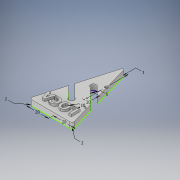
# Autodesk Inventor part: directional_arrow
Saved by Autodesk Inventor 2019 (Build 230136000, 136)
## iProperties
Created: 2019-04-03
Part Number: directional_arrow
Material: Generic
Document SubType Name: Modeling
Designer: jmc
Density: 1 g/cm^3
Appearance: Default
URL: https://www.amazon.es/MagiDeal-Marcador-Flecha-Triangular-Naufragios/dp/B07CHZN8H6
Author: jmc
Autodesk Inventor part; units mm, degrees
ref_plane "YZ Plane" through (0, 0, 0) normal (1, 0, 0) x (0, 1, 0)
ref_plane "XZ Plane" through (0, 0, 0) normal (0, 1, 0) x (-1, 0, 0)
ref_plane "XY Plane" through (0, 0, 0) normal (0, 0, 1) x (1, 0, 0)
sketch "Sketch1" plane through (0, 0, 0) normal (0, 1, 0) x (-1, 0, 0)
  line L0 (0, 0) -> (0, -40) construction
  line L1 (0, -40) -> (0, 29.0613) construction
  line L2 (0, 29.0613) -> (17.3386, 29.0613)
  line L3 (0, 29.0613) -> (-17.3386, 29.0613)
  arc A0 (19.2597, 26.505) -> (17.3386, 29.0613) centre (17.3386, 27.0613) ccw
  arc A1 (-17.3386, 29.0613) -> (-19.2597, 26.505) centre (-17.3386, 27.0613) ccw
  arc A2 (-0.9605, -36.6832) -> (0.9605, -36.6832) centre (0, -36.4051) ccw
  line L4 (0, 0) -> (0, 10) construction
  line L5 (0, 10) -> (0, -10) construction
  arc A3 (2.4749, 10.3536) -> (0, 7.5) centre (0, 10) ccw
  arc A4 (-1.7678, -11.7678) -> (0, -7.5) centre (0, -10) ccw
  line L6 (2.4749, 10.3536) -> (11.8634, 0.965)
  line L7 (-0.3536, 7.5251) -> (10.5931, -3.4215)
  line L8 (-1.7678, -11.7678) -> (-10.7883, -2.7472)
  line L9 (0.3536, -7.5251) -> (-13.3826, 6.211)
  line L10 (19.2597, 26.505) -> (11.8634, 0.965)
  line L11 (10.5931, -3.4215) -> (0.9605, -36.6832)
  line L12 (-19.2597, 26.505) -> (-13.3826, 6.211)
  line L13 (-10.7883, -2.7472) -> (-0.9605, -36.6832)
  line L14 (-14.9966, 24.7368) -> (15.142, 24.7368) construction
  line L15 (15.142, 24.7368) -> (15.142, 16.2798) construction
  line L16 (15.142, 16.2798) -> (-14.9966, 16.2798) construction
  line L17 (-14.9966, 16.2798) -> (-14.9966, 24.7368) construction
  line L18 (-8.7427, 16.4508) -> (-14.1549, 16.4508)
  line L19 (-14.1549, 16.4508) -> (-14.1549, 24.5658)
  line L20 (-14.1549, 24.5658) -> (-12.1162, 24.5658)
  line L21 (-12.1162, 24.5658) -> (-12.1162, 17.9962)
  line L22 (-12.1162, 17.9962) -> (-8.7427, 17.9962)
  line L23 (-8.7427, 17.9962) -> (-8.7427, 16.4508)
  spline S0 degree 2 poles (-0.3843, 20.5083) (-0.3843, 18.5354) (-2.4887, 16.2798) (-4.3169, 16.2798) knots 0 0 0 1 2 2 2
  spline S1 degree 2 poles (-4.3169, 16.2798) (-6.1517, 16.2798) (-8.2429, 18.5617) (-8.2429, 20.5083) knots 0 0 0 1 2 2 2
  spline S2 degree 2 poles (-8.2429, 20.5083) (-8.2429, 22.4614) (-6.1517, 24.7368) (-4.3169, 24.7368) knots 0 0 0 1 2 2 2
  spline S3 degree 2 poles (-4.3169, 24.7368) (-2.4887, 24.7368) (-0.3843, 22.4745) (-0.3843, 20.5083) knots 0 0 0 1 2 2 2
  spline S4 degree 2 poles (-2.4887, 20.5083) (-2.4887, 21.2382) (-2.7847, 22.2575) (-3.0411, 22.5798) knots 0 0 0 1 2 2 2
  spline S5 degree 2 poles (-3.0411, 22.5798) (-3.2976, 22.9151) (-3.9552, 23.2045) (-4.3103, 23.2045) knots 0 0 0 1 2 2 2
  spline S6 degree 2 poles (-4.3103, 23.2045) (-4.6852, 23.2045) (-5.2968, 22.9349) (-5.5795, 22.5929) knots 0 0 0 1 2 2 2
  spline S7 degree 2 poles (-5.5795, 22.5929) (-5.8294, 22.2773) (-6.1385, 21.2316) (-6.1385, 20.5083) knots 0 0 0 1 2 2 2
  spline S8 degree 2 poles (-6.1385, 20.5083) (-6.1385, 19.7586) (-5.8426, 18.7722) (-5.5861, 18.4368) knots 0 0 0 1 2 2 2
  spline S9 degree 2 poles (-5.5861, 18.4368) (-5.3296, 18.1014) (-4.6654, 17.812) (-4.3103, 17.812) knots 0 0 0 1 2 2 2
  spline S10 degree 2 poles (-4.3103, 17.812) (-3.9486, 17.812) (-3.2779, 18.1211) (-3.0345, 18.4499) knots 0 0 0 1 2 2 2
  spline S11 degree 2 poles (-3.0345, 18.4499) (-2.7715, 18.805) (-2.4887, 19.7454) (-2.4887, 20.5083) knots 0 0 0 1 2 2 2
  spline S12 degree 2 poles (4.3242, 16.2929) (2.496, 16.2929) (0.3522, 18.5025) (0.3522, 20.5017) knots 0 0 0 1 2 2 2
  spline S13 degree 2 poles (0.3522, 20.5017) (0.3522, 22.4285) (2.5026, 24.7236) (4.3308, 24.7236) knots 0 0 0 1 2 2 2
  spline S14 degree 2 poles (4.3308, 24.7236) (4.8108, 24.7236) (5.5868, 24.6118) (5.9419, 24.5197) knots 0 0 0 1 2 2 2
  spline S15 degree 2 poles (5.9419, 24.5197) (6.2181, 24.4342) (6.8692, 24.1515) (7.073, 24.0463) knots 0 0 0 1 2 2 2
  line L24 (7.073, 24.0463) -> (7.073, 22.1129)
  line L25 (7.073, 22.1129) -> (6.8692, 22.1129)
  spline S16 degree 2 poles (6.8692, 22.1129) (6.7179, 22.2444) (6.2707, 22.6126) (5.988, 22.7836) knots 0 0 0 1 2 2 2
  spline S17 degree 2 poles (5.988, 22.7836) (5.7052, 22.9612) (5.0278, 23.2045) (4.653, 23.2045) knots 0 0 0 1 2 2 2
  spline S18 degree 2 poles (4.653, 23.2045) (4.2124, 23.2045) (3.4824, 22.9283) (3.1471, 22.5798) knots 0 0 0 1 2 2 2
  spline S19 degree 2 poles (3.1471, 22.5798) (2.8446, 22.2707) (2.4566, 21.2119) (2.4566, 20.4951) knots 0 0 0 1 2 2 2
  spline S20 degree 2 poles (2.4566, 20.4951) (2.4566, 19.7389) (2.8577, 18.7064) (3.1865, 18.3907) knots 0 0 0 1 2 2 2
  spline S21 degree 2 poles (3.1865, 18.3907) (3.5022, 18.0817) (4.2782, 17.812) (4.6662, 17.812) knots 0 0 0 1 2 2 2
  spline S22 degree 2 poles (4.6662, 17.812) (5.0673, 17.812) (5.7973, 18.0817) (6.0472, 18.2461) knots 0 0 0 1 2 2 2
  spline S23 degree 2 poles (6.0472, 18.2461) (6.3233, 18.4105) (6.7376, 18.759) (6.8889, 18.8971) knots 0 0 0 1 2 2 2
  line L26 (6.8889, 18.8971) -> (7.073, 18.8971)
  line L27 (7.073, 18.8971) -> (7.073, 16.99)
  spline S24 degree 2 poles (7.073, 16.99) (6.8494, 16.8848) (6.2642, 16.6218) (5.9485, 16.5297) knots 0 0 0 1 2 2 2
  spline S25 degree 2 poles (5.9485, 16.5297) (5.5671, 16.4113) (4.9029, 16.2929) (4.3242, 16.2929) knots 0 0 0 1 2 2 2
  line L28 (7.4018, 16.4508) -> (10.1441, 24.5658)
  line L29 (10.1441, 24.5658) -> (12.3669, 24.5658)
  line L30 (12.3669, 24.5658) -> (15.1091, 16.4508)
  line L31 (15.1091, 16.4508) -> (13.0113, 16.4508)
  line L32 (13.0113, 16.4508) -> (12.505, 18.108)
  line L33 (12.505, 18.108) -> (9.9534, 18.108)
  line L34 (9.9534, 18.108) -> (9.4405, 16.4508)
  line L35 (9.4405, 16.4508) -> (7.4018, 16.4508)
  line L36 (12.0578, 19.581) -> (11.2292, 22.2641)
  line L37 (11.2292, 22.2641) -> (10.394, 19.581)
  line L38 (10.394, 19.581) -> (12.0578, 19.581)
  point P0 (20, 29.0613)
  point P1 (-20, 29.0613)
  dimension "d0" = 40
  dimension "d1" = 20
  dimension "d2" = 20
  dimension "d3" = 2
  dimension "d4" = 2
  dimension "d5" = 1
  dimension "d6" = 10
  dimension "d7" = 20
  dimension "d8" = 5
  dimension "d9" = 5
  constraints: 28 end point, 12 point on circle, 10 tangent, 7 point on line, 5 centre point, 2 coincident, 2 horizontal, 1 parallel, 1 vertical, 2 other
  measures "d0" distance of L0.start L0.end
  measures "d1" distance of L1.end point (20, 29.061)
  measures "d2" distance of L1.end point (-20, 29.061)
  measures "d3" radius of A0
  measures "d4" radius of A1
  measures "d5" radius of A2
  measures "d6" distance of L0.start L4.end
  measures "d7" distance of L4.end L5.end
  measures "d8" diameter of A3
  measures "d9" diameter of A4
extrude "Extrusion1" add sketch "Sketch1" along normal blind 5 contours L2 A0 L10 L6 A3 L7 L11 A2 L13 L8 A4 L9 L12 A1 L3 | L18 L19 L20 L21 L22 L23 | S0 S1 S2 S3 | S11 S10 S9 S8 S7 S6 S5 S4 | S12 S13 S14 S15 L24 L25 S16 S17 S18 S19 S20 S21 S22 S23 L26 L27 S24 S25 | L28 L29 L30 L31 L32 L33 L34 L35 | L38 L37 L36
extrude "Extrusion2" add sketch "Sketch1" along normal blind 7 contours L18 L19 L20 L21 L22 L23 | S0 S1 S2 S3 | S12 S13 S14 S15 L24 L25 S16 S17 S18 S19 S20 S21 S22 S23 L26 L27 S24 S25 | L28 L29 L30 L31 L32 L33 L34 L35
body "Solid1"
